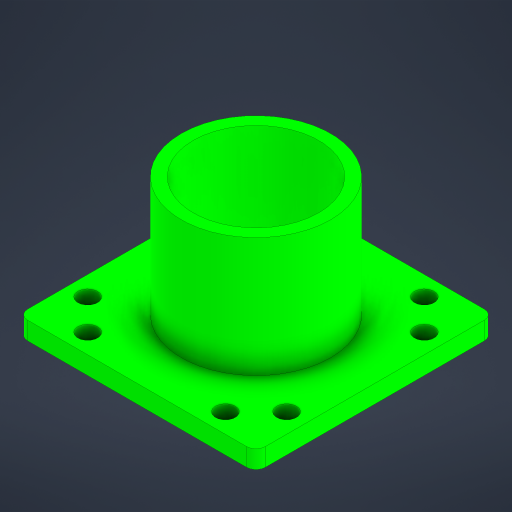
# Autodesk Inventor part: Flashlight Mount V1
Saved by Autodesk Inventor 2023.4 (Build 274418000, 418)
## iProperties
Created: 2022-07-25
Part Number: Flashlight Mount V1
Material: Generic
Document SubType Name: Modeling
Designer: xSibe
Density: 1 g/cm^3
Appearance: Plastic Red
Author: xSibe
Autodesk Inventor part; units mm, degrees
ref_plane "YZ Plane" through (0, 0, 0) normal (1, 0, 0) x (0, 1, 0)
ref_plane "XZ Plane" through (0, 0, 0) normal (0, 1, 0) x (-1, 0, 0)
ref_plane "XY Plane" through (0, 0, 0) normal (0, 0, 1) x (1, 0, 0)
sketch "Sketch1" plane through (0, 0, 0) normal (0, 1, 0) x (-1, 0, 0)
  circle A0 centre (20.8, -14.4) radius 2.0675
  circle A1 centre (14.4, -20.8) radius 2.0675
  circle A2 centre (20.8, 14.4) radius 13.125
  circle A3 centre (20.8, 14.4) radius 15.625
  circle A4 centre (-1.1, -7.5) radius 1.875 projected
  circle A5 centre (42.7, 36.3) radius 1.875 projected
  circle A6 centre (42.7, -7.5) radius 1.875 projected
  circle A7 centre (-1.1, 36.3) radius 1.875 projected
  circle A8 centre (35.2, 35.2) radius 2.0734 projected
  circle A9 centre (6.4, -6.4) radius 2.0734 projected
  circle A10 centre (35.2, -6.4) radius 2.0734 projected
  circle A11 centre (41.6, 0) radius 2.0734 projected
  line L0 (3.75, 31.45) -> (3.75, -2.65) projected
  line L1 (37.85, 31.45) -> (3.75, 31.45) projected
  line L2 (37.85, -2.65) -> (37.85, 31.45) projected
  line L3 (3.75, -2.65) -> (37.85, -2.65) projected
  circle A12 centre (41.6, 28.8) radius 2.0734 projected
  circle A13 centre (6.4, 35.2) radius 2.0734 projected
  circle A14 centre (0, 0) radius 2.0734 projected
  circle A15 centre (0, 28.8) radius 2.0734 projected
  line L4 (-2.1, 39.275) -> (43.7, 39.275) projected
  arc A16 (-2.1, 39.275) -> (-4.075, 37.3) centre (-2.1, 37.3) ccw projected
  line L5 (-4.075, -8.5) -> (-4.075, 37.3) projected
  arc A17 (-4.075, -8.5) -> (-2.1, -10.475) centre (-2.1, -8.5) ccw projected
  line L6 (43.7, -10.475) -> (-2.1, -10.475) projected
  arc A18 (43.7, -10.475) -> (45.675, -8.5) centre (43.7, -8.5) ccw projected
  line L7 (45.675, 37.3) -> (45.675, -8.5) projected
  arc A19 (45.675, 37.3) -> (43.7, 39.275) centre (43.7, 37.3) ccw projected
  line L8 (37.85, 14.4) -> (3.75, 14.4)
  dimension "d52" = 26.25
  dimension "d53" = 2.5
  constraints: 4 centre point, 3 midpoint, 2 end point, 1 coincident
  measures "d52" diameter of A2
  measures "d53" radial gap between concentric circles of A3 A2
extrude "Extrusion1" add sketch "Sketch1" along normal blind 3.75 contours L8 A3 A2 | A2 L8 A3 | L8 L2 L3 L0 A3 | A3 L8 L0 L1 L2 | A4 | A5 | A6 | A7 | A10 | A11 | L4 A19 L7 A18 L6 A17 L5 A16
extrude "Extrusion2" add sketch "Sketch1" along normal blind 25 from surface at 3.75 contours L8 A3 A2 | A2 L8 A3
sketch "Sketch2" plane through (0, 0, 0) normal (1, 0, 0) x (0, 1, 0)
  line L0 (3.75, 30.025) -> (3.75, -1.225) projected
  line L1 (28.75, 30.025) -> (28.75, -1.225) projected
  line L2 (28.75, 14.4) -> (3.75, 14.4)
  line L3 (28.75, 14.4) -> (16.25, 14.4)
  line L4 (28.75, 14.4) -> (22.5, 14.4)
  circle A0 centre (25.625, 14.4) radius 1.375
  circle A1 centre (20.875, 14.4) radius 1.375
  circle A2 centre (16.125, 14.4) radius 1.375
  circle A3 centre (11.375, 14.4) radius 1.375
  circle A4 centre (6.625, 14.4) radius 1.375
  point P0 (0, 0)
  dimension "d39" = 2.75
  dimension "d42" = 4.75
  constraints: 6 end point, 5 centre point, 5 midpoint, 1 horizontal, 8 other
  measures "d39" diameter of A0
  measures "d42" distance of A0.centre A1.centre
extrude "Extrusion3" cut sketch "Sketch2" along normal up to surface round surface about axis through (-20.8, 0, 14.4) along (0, 1, 0) radius 15.625 far side no
sketch "Sketch3" plane through (0, 0, 0) normal (0, -1, 0) x (1, 0, 0)
  circle A0 centre (-20.8, 14.4) radius 13.125 projected
  circle A1 centre (-20.8, 14.4) radius 10.625
  point P0 (0, 0)
  dimension "d49" = 2.5
  constraints: 1 centre point
  measures "d49" radial gap between concentric circles of A0 A1
extrude "Extrusion4" add sketch "Sketch3" against normal blind 2.5
body "Solid1"
